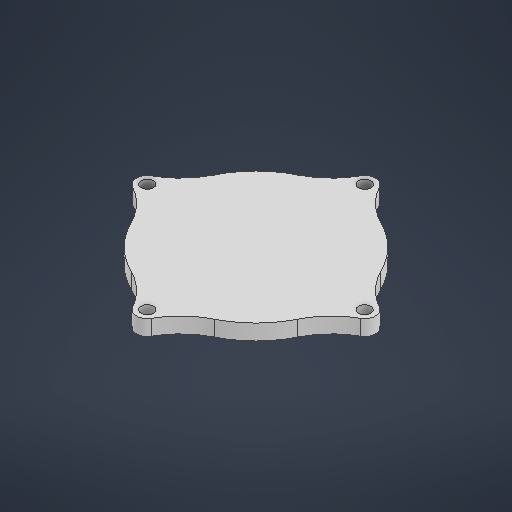
# Autodesk Inventor part: tapa
Saved by Autodesk Inventor 2025.3 (Build 293356000, 356)
## iProperties
Created: 2025-10-20
Part Number: tapa
Material: Generic
Document SubType Name: Modeling
Designer: sophi
Density: 1 g/cm^3
Appearance: Default
Author: sophi
Autodesk Inventor part; units mm, degrees
ref_plane "YZ Plane" through (0, 0, 0) normal (1, 0, 0) x (0, 1, 0)
ref_plane "XZ Plane" through (0, 0, 0) normal (0, 1, 0) x (-1, 0, 0)
ref_plane "XY Plane" through (0, 0, 0) normal (0, 0, 1) x (1, 0, 0)
sketch "Sketch1" plane through (0, 0, 0) normal (0, 1, 0) x (-1, 0, 0)
  circle A0 centre (0, 0) radius 30
  circle A1 centre (0, 0) radius 27.5
  circle A2 centre (0, 35) radius 3.5
  circle A3 centre (0, 35) radius 2
  arc A4 (3.0597, 36.6995) -> (13.3557, 26.8631) centre (24.0402, 48.3536) ccw
  arc A5 (-13.3557, 26.8631) -> (-3.0597, 36.6995) centre (-24.0402, 48.3536) ccw
  arc A6 (-36.6995, 3.0597) -> (-26.8631, 13.3557) centre (-48.3536, 24.0402) ccw
  circle A7 centre (-35, 0) radius 3.5
  circle A8 centre (-35, 0) radius 2
  arc A9 (-26.8631, -13.3557) -> (-36.6995, -3.0597) centre (-48.3536, -24.0402) ccw
  arc A10 (-3.0597, -36.6995) -> (-13.3557, -26.8631) centre (-24.0402, -48.3536) ccw
  circle A11 centre (0, -35) radius 3.5
  circle A12 centre (0, -35) radius 2
  arc A13 (13.3557, -26.8631) -> (3.0597, -36.6995) centre (24.0402, -48.3536) ccw
  arc A14 (36.6995, -3.0597) -> (26.8631, -13.3557) centre (48.3536, -24.0402) ccw
  circle A15 centre (35, 0) radius 3.5
  circle A16 centre (35, 0) radius 2
  arc A17 (26.8631, 13.3557) -> (36.6995, 3.0597) centre (48.3536, 24.0402) ccw
  point P0 (26.8631, 13.3557)
  point P1 (-26.8631, 13.3557)
  point P2 (-26.8631, -13.3557)
  point P3 (-13.3557, -26.8631)
  point P4 (13.3557, -26.8631)
  point P5 (26.8631, -13.3557)
  dimension "d0" = 60
  dimension "d1" = 55
  dimension "d2" = 7
  dimension "d3" = 4
  dimension "d4" = 35
  dimension "d5" = 24
  dimension "d8" = 360
  constraints: 26 point on circle, 18 centre point, 6 coincident, 4 tangent, 1 equal radius, 1 vertical alignment, 49 other
  measures "d0" diameter of A0
  measures "d1" diameter of A1
  measures "d2" diameter of A2
  measures "d3" diameter of A3
  measures "d4" distance of point (0, 0) A2.centre
  measures "d5" radius of A4
extrude "Extrusion1" add sketch "Sketch1" along normal blind 5 contours A0 | A0 A17 A15 A14 | A0 A5 A2 A4 | A15 | A13 A11 A10 A0 | A2 | A11 | A0 A9 A7 A6 | A7 | A1
body "Solid1"
